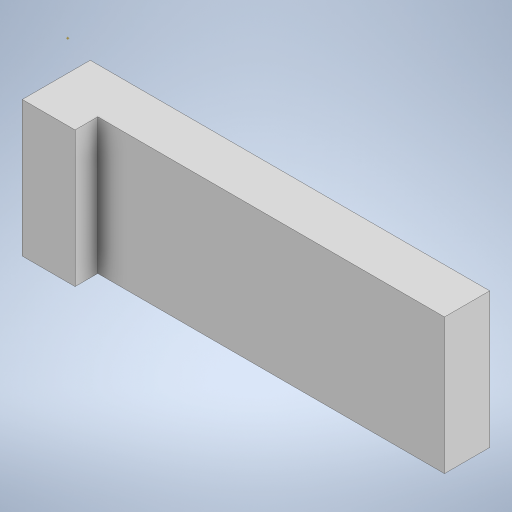
# Autodesk Inventor part: ServerCabinetRight
Saved by Autodesk Inventor 2023.1 (Build 271208000, 208)
## iProperties
Created: 2023-06-06
Part Number: ServerCabinetRight
Material: Generic
Document SubType Name: Modeling
Designer: rwc6
Density: 1 g/cm^3
Appearance: Default
Author: rwc6
Autodesk Inventor part; units mm, degrees
ref_plane "YZ Plane" through (0, 0, 0) normal (1, 0, 0) x (0, 1, 0)
ref_plane "XZ Plane" through (0, 0, 0) normal (0, 1, 0) x (-1, 0, 0)
ref_plane "XY Plane" through (0, 0, 0) normal (0, 0, 1) x (1, 0, 0)
sketch "Sketch1" plane through (0, 0, 0) normal (1, 0, 0) x (0, 1, 0)
  line L0 (-900, 300) -> (900, 300)
  line L1 (900, 300) -> (900, -300)
  line L2 (900, -300) -> (-900, -300)
  line L3 (-900, -300) -> (-900, 300)
  line L4 (-900, 300) -> (900, -300) construction
  line L5 (900, 300) -> (-900, -300) construction
  point P0 (0, 0)
  dimension "d0" = 1800
  dimension "d1" = 600
  constraints: 12 end point, 2 midpoint, 2 parallel, 1 horizontal, 1 perpendicular
  measures "d0" distance of L1.end L2.end
  measures "d1" distance of L0.end L1.end
extrude "Extrusion1" add sketch "Sketch1" against normal blind 5300
sketch "Sketch2" plane through (0, -900, -300) normal (0, 0, -1) x (-1, 0, 0)
  line L0 (0, 1800) -> (5300, 1800) projected
  line L1 (5300, 1800) -> (4600, 1800)
  line L2 (4600, 1800) -> (4600, 0)
  line L3 (4600, 0) -> (5300, 0)
  line L4 (5300, 0) -> (5300, 1800)
  point P0 (0, 900)
  dimension "d4" = 700
  constraints: 8 end point, 2 parallel, 1 horizontal, 1 perpendicular
  measures "d4" distance of L3.end L2.end
extrude "Extrusion2" add sketch "Sketch2" along normal blind 301.625
sketch "Sketch3" plane through (0, -900, -601.625) normal (0, 0, -1) x (-1, 0, 0)
  line L0 (5300, 1800) -> (4600, 1800) projected
  line L1 (4600, 1800) -> (4600, 0) projected
  line L2 (4600, 0) -> (5300, 0) projected
  line L3 (5300, 0) -> (5300, 1800) projected
  point P0 (0, 900)
extrude "Extrusion3" cut sketch "Sketch3" against normal up to surface (301.625 mm away)
sketch "Sketch4" plane through (0, -900, 300) normal (0, 0, 1) x (1, 0, 0)
  line L0 (0, 0) -> (-5300, 0) projected
  line L1 (-5300, 0) -> (-4600, 0)
  line L2 (-4600, 0) -> (-4600, 1800)
  line L3 (-4600, 1800) -> (-5300, 1800)
  line L4 (-5300, 1800) -> (-5300, 0)
  point P0 (0, 900)
  point P1 (-4600, 0)
  dimension "d9" = 700
  dimension "d10" = 1800
  constraints: 8 end point, 2 parallel, 1 horizontal, 1 perpendicular
  measures "d9" distance of L3.end L2.end
  measures "d10" distance of L2.end L1.end
extrude "Extrusion4" add sketch "Sketch4" along normal blind 301.625
sketch "Sketch6" plane through (-5300, 0, 0) normal (-1, 0, 0) x (0, 0, 1)
  line L0 (-300, -900) -> (-300, 900) construction
  line L1 (-300, 900) -> (0, 900) construction
  line L2 (300, 900) -> (300, -900) construction
  line L3 (-300, 900) -> (0, 900) construction
  line L4 (0, 900) -> (0, 1301.6) construction
  point P0 (0, 0)
  dimension "d14" = 300
  dimension "d15" = 0
  dimension "d16" = 401.6
  dimension "d17" = 90
  constraints: 6 end point, 2 perpendicular, 1 collinear, 1 horizontal
  measures "d14" distance of L0.end L1.end
  measures "d15" distance between parallel lines of L1 L3
  measures "d16" distance of L1.end L4.end
  measures "d17" angle of L4 L1
equation "\"d0\" = serv_h"
equation "\"d1\" = serv_w"
equation "\"d2\" = serv_e"
equation "\"d14\" = 0.5 * serv_w"
equation "\"d16\" = tray_h + leg_e"
equation "\"serv_h\" = 1800"
equation "\"serv_w\" = 600"
equation "\"serv_e\" = 5300"
equation "\"tray_h\" = 101.6"
equation "\"leg_e\" = 300"
